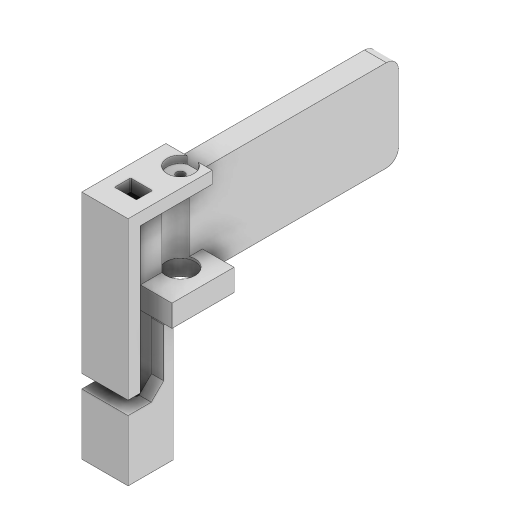
# Autodesk Inventor part: OT2-Gripper V1-1 BG Layout
Saved by Autodesk Inventor 2024.3 (Build 283343000, 343)
## iProperties
Created: 2024-09-11
Part Number: OT2-Gripper V1-1 BG Layout
Material: Generisch
Document SubType Name: Modeling
Designer: Martin
Density: 1 g/cm^3
Appearance: Vorgabe
Author: Martin
Autodesk Inventor part; units mm, degrees
ref_plane "XZ Plane" through (0, 0, 0) normal (0, 1, 0) x (-1, 0, 0)
ref_plane "XY Plane" through (0, 0, 0) normal (0, 0, 1) x (1, 0, 0)
sketch "OT2-Interface-blk" plane through (0, 0, 0) normal (0, 0, 1) x (1, 0, 0)
  circle A0 centre (25.0589, -118.2387) radius 1.5 construction
  circle A1 centre (25.0589, -91.7387) radius 1.5 construction
  circle A2 centre (-63.9411, -118.2387) radius 1.5 construction
  line L0 (32.0589, -86.2387) -> (-73.9411, -86.2387) construction
  line L1 (-73.9411, -86.2387) -> (-73.9411, -123.7387) construction
  line L2 (-73.9411, -123.7387) -> (32.0589, -123.7387) construction
  line L3 (32.0589, -123.7387) -> (32.0589, -86.2387) construction
  point P0 (-34.6142, -114.104)
  dimension "d0" = 37.5
  dimension "d1" = 26.5
  dimension "d2" = 3
  dimension "d3" = 5.5
  dimension "d4" = 7
  dimension "d5" = 89
  dimension "d6" = 106
  measures "d0" distance of L2.end L0.start
  measures "d1" distance of A0.centre A1.centre
  measures "d2" diameter of A0
  measures "d3" distance from line of L0 A1.centre
  measures "d4" distance from line of L3 A1.centre
  measures "d5" distance of A2.centre A0.centre
  measures "d6" distance of L0.start L0.end
sketch "NEMA08-04LA captive linear actor-blk" plane through (0, 0, 0) normal (0, 0, 1) x (1, 0, 0)
  line L0 (156.7218, 142.634) -> (136.7218, 142.634)
  line L1 (136.7218, 142.634) -> (136.7218, 170.634)
  line L2 (136.7218, 170.634) -> (156.7218, 170.634)
  line L3 (156.7218, 170.634) -> (156.7218, 142.634)
  line L4 (154.7218, 170.634) -> (138.7218, 170.634)
  line L5 (138.7218, 170.634) -> (138.7218, 172.134)
  line L6 (138.7218, 172.134) -> (154.7218, 172.134)
  line L7 (154.7218, 172.134) -> (154.7218, 170.634)
  line L8 (148.2218, 248.634) -> (145.2218, 248.634) construction
  line L9 (145.2218, 248.634) -> (145.2218, 252.634) construction
  line L10 (145.2218, 252.634) -> (148.2218, 252.634) construction
  line L11 (148.2218, 252.634) -> (148.2218, 248.634) construction
  line L12 (149.9718, 210.634) -> (143.4718, 210.634)
  line L13 (143.4718, 210.634) -> (143.4718, 248.634) construction
  line L14 (143.4718, 248.634) -> (149.9718, 248.634) construction
  line L15 (149.9718, 248.634) -> (149.9718, 210.634) construction
  line L16 (148.7218, 142.634) -> (144.7218, 142.634) construction
  line L17 (144.7218, 142.634) -> (144.7218, 115.634) construction
  line L18 (144.7218, 115.634) -> (148.7218, 115.634) construction
  line L19 (148.7218, 115.634) -> (148.7218, 142.634) construction
  line L20 (146.7218, 115.634) -> (146.7218, 252.634)
  line L21 (153.2218, 172.134) -> (140.2218, 172.134)
  line L22 (140.2218, 172.134) -> (140.2218, 178.134)
  line L23 (140.2218, 178.134) -> (153.2218, 178.134)
  line L24 (153.2218, 178.134) -> (153.2218, 172.134)
  line L25 (151.7218, 178.134) -> (141.7218, 178.134)
  line L26 (141.7218, 178.134) -> (141.7218, 210.634)
  line L27 (141.7218, 210.634) -> (151.7218, 210.634)
  line L28 (151.7218, 210.634) -> (151.7218, 178.134)
  line L29 (148.2218, 210.634) -> (145.2218, 210.634)
  line L30 (145.2218, 210.634) -> (145.2218, 214.634)
  line L31 (145.2218, 214.634) -> (148.2218, 214.634)
  line L32 (148.2218, 214.634) -> (148.2218, 210.634)
  line L33 (156.7218, 460.634) -> (136.7218, 460.634)
  line L34 (136.7218, 460.634) -> (136.7218, 480.634)
  line L35 (136.7218, 480.634) -> (156.7218, 480.634)
  line L36 (156.7218, 480.634) -> (156.7218, 460.634)
  circle A0 centre (154.7218, 462.634) radius 1 construction
  circle A1 centre (154.7218, 478.634) radius 1 construction
  circle A2 centre (138.7218, 478.634) radius 1 construction
  circle A3 centre (138.7218, 462.634) radius 1 construction
  circle A4 centre (146.7218, 470.634) radius 6.5
  circle A5 centre (146.7218, 470.634) radius 5
  circle A6 centre (146.7218, 470.634) radius 3.25 construction
  circle A7 centre (146.7218, 470.634) radius 1.5
  circle A8 centre (146.7218, 470.634) radius 2 construction
  circle A9 centre (146.7218, 470.634) radius 8
  line L37 (154.7218, 170.634) -> (154.7218, 167.634) construction
  line L38 (138.7218, 170.634) -> (138.7218, 167.634) construction
  point P0 (146.7218, 170.634)
  point P1 (146.7218, 210.634)
  point P2 (146.7218, 172.134)
  point P3 (146.7218, 178.134)
  point P4 (146.7218, 214.634)
  point P5 (146.7218, 480.634)
  point P6 (156.7218, 470.634)
  dimension "d9" = 4
  dimension "d10" = 16
  dimension "d11" = 1.5
  dimension "d12" = 7.5
  dimension "d14" = 3
  dimension "d15" = 6.5
  dimension "d16" = 40
  dimension "d17" = 10
  dimension "d18" = 38
  dimension "d19" = 20
  dimension "d20" = 28
  dimension "d21" = 4
  dimension "d22" = 27
  dimension "d23" = 2
  dimension "d24" = 16
  dimension "d25" = 16
  dimension "d26" = 2
  dimension "d27" = 2
  dimension "d28" = 300
  dimension "d29" = 3
  dimension "d30" = 13
  measures "d9" distance of L10.end L8.start
  measures "d10" distance of L4.start L4.end
  measures "d11" distance of L6.end L4.start
  measures "d12" distance between parallel lines of L2 L23
  measures "d14" distance of L9.end L10.end
  measures "d15" distance between parallel lines of L13 L15
  measures "d16" distance between parallel lines of L2 L27
  measures "d17" distance between parallel lines of L26 L28
  measures "d18" distance between parallel lines of L27 L14
  measures "d19" distance of L1.end L2.end
  measures "d20" distance of L2.end L0.start
  measures "d21" distance of L17.end L18.end
  measures "d22" distance of L18.end L16.start
  measures "d23" diameter of A1
  measures "d24" distance of A1.centre A0.centre
  measures "d25" distance of A1.centre A2.centre
  measures "d26" distance from line of L36 A1.centre
  measures "d27" distance from line of A1.centre L35
  measures "d28" distance from line of L2 A4.centre
  measures "d29" distance of L37.start L37.end
  measures "d30" distance between parallel lines of L22 L24
sketch "linear gudance Type10mm-blk" plane through (0, 0, 0) normal (0, 0, 1) x (1, 0, 0)
  line L0 (-133.9665, -98.7965) -> (-140.5665, -98.7965)
  line L1 (-140.5665, -98.7965) -> (-140.5665, -3.7965)
  line L2 (-140.5665, -3.7965) -> (-133.9665, -3.7965)
  line L3 (-133.9665, -3.7965) -> (-133.9665, -98.7965)
  line L4 (-135.3665, -71.2965) -> (-143.9665, -71.2965)
  line L5 (-143.9665, -71.2965) -> (-143.9665, -31.2965)
  line L6 (-143.9665, -31.2965) -> (-135.3665, -31.2965)
  line L7 (-135.3665, -31.2965) -> (-135.3665, -71.2965)
  line L8 (-135.3665, 238.7035) -> (-143.9665, 238.7035)
  line L9 (-143.9665, 238.7035) -> (-143.9665, 258.7035)
  line L10 (-143.9665, 258.7035) -> (-135.3665, 258.7035)
  line L11 (-135.3665, 258.7035) -> (-135.3665, 238.7035)
  line L12 (-133.9665, 244.2035) -> (-140.5665, 244.2035)
  line L13 (-140.5665, 244.2035) -> (-140.5665, 253.2035)
  line L14 (-140.5665, 253.2035) -> (-133.9665, 253.2035)
  line L15 (-133.9665, 253.2035) -> (-133.9665, 244.2035)
  line L16 (-423.9665, -71.2965) -> (-443.9665, -71.2965)
  line L17 (-443.9665, -71.2965) -> (-443.9665, -31.2965)
  line L18 (-443.9665, -31.2965) -> (-423.9665, -31.2965)
  line L19 (-423.9665, -31.2965) -> (-423.9665, -71.2965)
  line L20 (-429.4665, -98.7965) -> (-438.4665, -98.7965)
  line L21 (-438.4665, -98.7965) -> (-438.4665, -3.7965)
  line L22 (-438.4665, -3.7965) -> (-429.4665, -3.7965)
  line L23 (-429.4665, -3.7965) -> (-429.4665, -98.7965)
  line L24 (-433.9665, -98.7965) -> (-433.9665, -3.7965) construction
  line L25 (-135.3665, 248.7035) -> (-140.5665, 248.7035) construction
  line L26 (-133.9665, -91.2965) -> (-140.5665, -91.2965) construction
  line L27 (-136.5665, -94.2965) -> (-136.5665, -88.2965) construction
  line L28 (-136.5665, -89.4965) -> (-133.9665, -89.4965) construction
  line L29 (-133.9665, -93.0965) -> (-136.5665, -93.0965) construction
  line L30 (-136.5665, -94.2965) -> (-140.5665, -94.2965) construction
  line L31 (-136.5665, -88.2965) -> (-140.5665, -88.2965) construction
  line L32 (-136.5665, -69.4965) -> (-133.9665, -69.4965) construction
  line L33 (-133.9665, -73.0965) -> (-136.5665, -73.0965) construction
  line L34 (-136.5665, -74.2965) -> (-136.5665, -68.2965) construction
  line L35 (-133.9665, -71.2965) -> (-140.5665, -71.2965) construction
  line L36 (-136.5665, -74.2965) -> (-140.5665, -74.2965) construction
  line L37 (-136.5665, -68.2965) -> (-140.5665, -68.2965) construction
  line L38 (-136.5665, -49.4965) -> (-133.9665, -49.4965) construction
  line L39 (-133.9665, -53.0965) -> (-136.5665, -53.0965) construction
  line L40 (-136.5665, -54.2965) -> (-136.5665, -48.2965) construction
  line L41 (-133.9665, -51.2965) -> (-140.5665, -51.2965) construction
  line L42 (-136.5665, -54.2965) -> (-140.5665, -54.2965) construction
  line L43 (-136.5665, -48.2965) -> (-140.5665, -48.2965) construction
  line L44 (-136.5665, -29.4965) -> (-133.9665, -29.4965) construction
  line L45 (-133.9665, -33.0965) -> (-136.5665, -33.0965) construction
  line L46 (-136.5665, -34.2965) -> (-136.5665, -28.2965) construction
  line L47 (-133.9665, -31.2965) -> (-140.5665, -31.2965) construction
  line L48 (-136.5665, -34.2965) -> (-140.5665, -34.2965) construction
  line L49 (-136.5665, -28.2965) -> (-140.5665, -28.2965) construction
  line L50 (-136.5665, -9.4965) -> (-133.9665, -9.4965) construction
  line L51 (-133.9665, -13.0965) -> (-136.5665, -13.0965) construction
  line L52 (-136.5665, -14.2965) -> (-136.5665, -8.2965) construction
  line L53 (-133.9665, -11.2965) -> (-140.5665, -11.2965) construction
  line L54 (-136.5665, -14.2965) -> (-140.5665, -14.2965) construction
  line L55 (-136.5665, -8.2965) -> (-140.5665, -8.2965) construction
  circle A0 centre (-433.9665, -91.2965) radius 3 construction
  circle A1 centre (-433.9665, -91.2965) radius 1.8 construction
  circle A2 centre (-433.9665, -71.2965) radius 1.8 construction
  circle A3 centre (-433.9665, -71.2965) radius 3 construction
  circle A4 centre (-433.9665, -51.2965) radius 1.8 construction
  circle A5 centre (-433.9665, -51.2965) radius 3 construction
  circle A6 centre (-433.9665, -31.2965) radius 1.8 construction
  circle A7 centre (-433.9665, -31.2965) radius 3 construction
  circle A8 centre (-433.9665, -11.2965) radius 1.8 construction
  circle A9 centre (-433.9665, -11.2965) radius 3 construction
  line L56 (-140.5665, 245.7035) -> (-136.5665, 245.7035) construction
  line L57 (-136.5665, 245.7035) -> (-136.5665, 251.7035) construction
  line L58 (-136.5665, 251.7035) -> (-140.5665, 251.7035) construction
  line L59 (-136.5665, 250.5035) -> (-133.9665, 250.5035) construction
  line L60 (-133.9665, 246.9035) -> (-136.5665, 246.9035) construction
  line L61 (-143.9665, 241.2035) -> (-139.9665, 241.2035) construction
  line L62 (-143.9665, 256.2035) -> (-139.9665, 256.2035) construction
  line L63 (-143.9665, -59.2965) -> (-139.9665, -59.2965) construction
  line L64 (-143.9665, -43.2965) -> (-139.9665, -43.2965) construction
  circle A10 centre (-426.4665, -59.2965) radius 1.5 construction
  circle A11 centre (-426.4665, -43.2965) radius 1.5 construction
  circle A12 centre (-441.4665, -59.2965) radius 1.5 construction
  circle A13 centre (-441.4665, -43.2965) radius 1.5 construction
  point P0 (-136.5665, -91.2965)
  point P1 (-136.5665, -71.2965)
  point P2 (-136.5665, -51.2965)
  point P3 (-136.5665, -31.2965)
  point P4 (-136.5665, -11.2965)
  point P5 (-135.3665, -51.2965)
  point P6 (-433.9665, -31.2965)
  dimension "LgGuideHolePitch" = 20
  dimension "LgGuideLength" = 95
  dimension "LgGuideHoleDm2" = 3.6
  dimension "LgGuideHoleDm1" = 6
  dimension "LgGuideHoleDm1Depth" = 4
  dimension "LgGuideHeigth" = 6.6
  dimension "LgSystemHeigth" = 10
  dimension "LgStageHeigth" = 8.6
  dimension "LgStageLength" = 40
  dimension "LgGuideWidth" = 9
  dimension "LgStageWidth" = 20
  dimension "d48" = 300
  dimension "d49" = 300
  dimension "d52" = 20
  dimension "d57" = 3.6
  dimension "LgStageHolePitchX" = 15
  dimension "LgStageHolePitchZ" = 16
  dimension "d60" = 15
  dimension "LgStageHoleDepth" = 4
  dimension "LgStageHoleDm" = 3
  measures "LgGuideHolePitch" distance of L28.end L32.end
  measures "LgGuideLength" distance of L2.end L0.start
  measures "LgGuideHoleDm2" distance between parallel lines of L28 L29
  measures "LgGuideHoleDm1" distance of L27.start L27.end
  measures "LgGuideHoleDm1Depth" distance of L27.end L31.end
  measures "LgGuideHeigth" distance of L0.start L0.end
  measures "LgSystemHeigth" distance between parallel lines of L5 L3
  measures "LgStageHeigth" distance of L4.start L4.end
  measures "LgStageLength" distance of L4.end L5.end
  measures "LgGuideWidth" distance of L14.end L12.start
  measures "LgStageWidth" distance of L8.end L9.end
  measures "d48" distance from line of L41.start L25
  measures "d49" distance between parallel lines of L3 L24
  measures "d52" distance of A1.centre A2.centre
  measures "d57" distance between parallel lines of L59 L60
  measures "LgStageHolePitchX" distance between parallel lines of L62 L61
  measures "LgStageHolePitchZ" distance between parallel lines of L64 L63
  measures "d60" distance of point (-441.466, -43.296) point (-426.466, -43.296)
  measures "LgStageHoleDepth" distance of L63.start L63.end
  measures "LgStageHoleDm" diameter of A10
sketch "Skizze1" plane through (0, 0, 0) normal (1, 0, 0) x (0, 1, 0)
  line L0 (48, -18.75) -> (-53, -18.75)
  line L1 (-53, -18.75) -> (-53, 18.75)
  line L2 (-53, 18.75) -> (48, 18.75)
  line L3 (53, 13.75) -> (53, -13.75)
  arc A0 (53, 13.75) -> (48, 18.75) centre (48, 13.75) ccw
  arc A1 (48, -18.75) -> (53, -13.75) centre (48, -13.75) ccw
  circle A2 centre (46, 13.25) radius 2.05
  circle A3 centre (46, -13.25) radius 2.05
  circle A4 centre (-43, -13.25) radius 2.05
  line L4 (-49.5, -68.75) -> (-68, -68.75)
  line L5 (-68, -68.75) -> (-68, -43.75)
  line L6 (-68, -43.75) -> (-49.5, -43.75)
  line L7 (-49.5, -43.75) -> (-49.5, -68.75)
  line L8 (-49.5, -43.75) -> (-53.4, -43.75)
  line L9 (-53.4, -43.75) -> (-53.4, -18.75)
  line L10 (-53.4, -18.75) -> (-49.5, -18.75)
  line L11 (-49.5, -18.75) -> (-49.5, -43.75)
  line L12 (-63, -38.25) -> (-68, -38.25)
  line L13 (-68, -38.25) -> (-68, 21.25)
  line L14 (-68, 21.25) -> (-63, 21.25)
  line L15 (-63, 21.25) -> (-63, -38.25)
  line L16 (-68, 21.25) -> (-33.5, 21.25)
  line L17 (-33.5, 21.25) -> (-33.5, 26.25)
  line L18 (-33.5, 26.25) -> (-68, 26.25)
  line L19 (-68, 26.25) -> (-68, 21.25)
  line L20 (-63, 1.75) -> (-68, 1.75) construction
  line L21 (-65.5, 1.75) -> (-65.5, -38.25) construction
  line L22 (-27.5, -18.75) -> (-27.5, -9.75)
  line L23 (-27.5, -9.75) -> (-53, -9.75)
  line L24 (-38.5, -18.75) -> (-30.5, -18.75)
  line L25 (-30.5, -18.75) -> (-30.5, -9.75)
  line L26 (-30.5, -9.75) -> (-38.5, -9.75)
  line L27 (-38.5, -9.75) -> (-38.5, -18.75)
  line L28 (-65.5, -26.25) -> (-68, -26.25) construction
  line L29 (-65.5, -10.25) -> (-68, -10.25) construction
  line L30 (-53.4, -38.6642) -> (-58.4858, -43.75)
  line L31 (-63, -38.25) -> (-54.4, -38.25) construction
  line L32 (-54.4, -38.25) -> (-54.4, -27.75) construction
  circle A5 centre (-54.4, -38.25) radius 1 construction
  circle A6 centre (46, -13.25) radius 1.5 construction
  circle A7 centre (46, 13.25) radius 1.5 construction
  circle A8 centre (-43, -13.25) radius 1.5 construction
  line L33 (53, 18.75) -> (-53, 18.75) construction
  line L34 (-53, 18.75) -> (-53, -18.75) construction
  line L35 (-53, -18.75) -> (53, -18.75) construction
  line L36 (53, -18.75) -> (53, 18.75) construction
  line L37 (-28.5, -46.75) -> (-48.5, -46.75)
  line L38 (-48.5, -46.75) -> (-48.5, -18.75)
  line L39 (-48.5, -18.75) -> (-28.5, -18.75)
  line L40 (-28.5, -18.75) -> (-28.5, -46.75)
  line L41 (-30.5, -18.75) -> (-46.5, -18.75)
  line L42 (-46.5, -18.75) -> (-46.5, -17.25)
  line L43 (-46.5, -17.25) -> (-30.5, -17.25)
  line L44 (-30.5, -17.25) -> (-30.5, -18.75)
  line L45 (-37, 59.25) -> (-40, 59.25) construction
  line L46 (-40, 59.25) -> (-40, 63.25) construction
  line L47 (-40, 63.25) -> (-37, 63.25) construction
  line L48 (-37, 63.25) -> (-37, 59.25) construction
  line L49 (-35.25, 21.25) -> (-41.75, 21.25)
  line L50 (-41.75, 21.25) -> (-41.75, 59.25) construction
  line L51 (-41.75, 59.25) -> (-35.25, 59.25) construction
  line L52 (-35.25, 59.25) -> (-35.25, 21.25) construction
  line L53 (-36.5, -46.75) -> (-40.5, -46.75) construction
  line L54 (-40.5, -46.75) -> (-40.5, -73.75) construction
  line L55 (-40.5, -73.75) -> (-36.5, -73.75) construction
  line L56 (-36.5, -73.75) -> (-36.5, -46.75) construction
  line L57 (-38.5, -73.75) -> (-38.5, 63.25)
  line L58 (-32, -17.25) -> (-45, -17.25)
  line L59 (-45, -17.25) -> (-45, -11.25)
  line L60 (-45, -11.25) -> (-32, -11.25)
  line L61 (-32, -11.25) -> (-32, -17.25)
  line L62 (-33.5, -11.25) -> (-43.5, -11.25)
  line L63 (-43.5, -11.25) -> (-43.5, 21.25)
  line L64 (-43.5, 21.25) -> (-33.5, 21.25)
  line L65 (-33.5, 21.25) -> (-33.5, -11.25)
  line L66 (-37, 21.25) -> (-40, 21.25)
  line L67 (-40, 21.25) -> (-40, 25.25)
  line L68 (-40, 25.25) -> (-37, 25.25)
  line L69 (-37, 25.25) -> (-37, 21.25)
  line L70 (-28.5, 271.25) -> (-48.5, 271.25)
  line L71 (-48.5, 271.25) -> (-48.5, 291.25)
  line L72 (-48.5, 291.25) -> (-28.5, 291.25)
  line L73 (-28.5, 291.25) -> (-28.5, 271.25)
  circle A9 centre (-30.5, 273.25) radius 1 construction
  circle A10 centre (-30.5, 289.25) radius 1 construction
  circle A11 centre (-46.5, 289.25) radius 1 construction
  circle A12 centre (-46.5, 273.25) radius 1 construction
  circle A13 centre (-38.5, 281.25) radius 6.5
  circle A14 centre (-38.5, 281.25) radius 5
  circle A15 centre (-38.5, 281.25) radius 3.25 construction
  circle A16 centre (-38.5, 281.25) radius 1.5
  circle A17 centre (-38.5, 281.25) radius 2 construction
  circle A18 centre (-38.5, 281.25) radius 8
  line L74 (-30.5, -18.75) -> (-30.5, -21.75) construction
  line L75 (-46.5, -18.75) -> (-46.5, -21.75) construction
  line L76 (-53, -55.25) -> (-59.6, -55.25)
  line L77 (-59.6, -55.25) -> (-59.6, 39.75)
  line L78 (-59.6, 39.75) -> (-53, 39.75)
  line L79 (-53, 39.75) -> (-53, -55.25)
  line L80 (-54.4, -27.75) -> (-63, -27.75)
  line L81 (-63, -27.75) -> (-63, 12.25)
  line L82 (-63, 12.25) -> (-54.4, 12.25)
  line L83 (-54.4, 12.25) -> (-54.4, -27.75)
  line L84 (-54.4, 282.25) -> (-63, 282.25)
  line L85 (-63, 282.25) -> (-63, 302.25)
  line L86 (-63, 302.25) -> (-54.4, 302.25)
  line L87 (-54.4, 302.25) -> (-54.4, 282.25)
  line L88 (-53, 287.75) -> (-59.6, 287.75)
  line L89 (-59.6, 287.75) -> (-59.6, 296.75)
  line L90 (-59.6, 296.75) -> (-53, 296.75)
  line L91 (-53, 296.75) -> (-53, 287.75)
  line L92 (-343, -27.75) -> (-363, -27.75)
  line L93 (-363, -27.75) -> (-363, 12.25)
  line L94 (-363, 12.25) -> (-343, 12.25)
  line L95 (-343, 12.25) -> (-343, -27.75)
  line L96 (-348.5, -55.25) -> (-357.5, -55.25)
  line L97 (-357.5, -55.25) -> (-357.5, 39.75)
  line L98 (-357.5, 39.75) -> (-348.5, 39.75)
  line L99 (-348.5, 39.75) -> (-348.5, -55.25)
  line L100 (-353, -55.25) -> (-353, 39.75) construction
  line L101 (-54.4, 292.25) -> (-59.6, 292.25) construction
  line L102 (-53, -47.75) -> (-59.6, -47.75) construction
  line L103 (-55.6, -50.75) -> (-55.6, -44.75) construction
  line L104 (-55.6, -45.95) -> (-53, -45.95) construction
  line L105 (-53, -49.55) -> (-55.6, -49.55) construction
  line L106 (-55.6, -50.75) -> (-59.6, -50.75) construction
  line L107 (-55.6, -44.75) -> (-59.6, -44.75) construction
  line L108 (-55.6, -25.95) -> (-53, -25.95) construction
  line L109 (-53, -29.55) -> (-55.6, -29.55) construction
  line L110 (-55.6, -30.75) -> (-55.6, -24.75) construction
  line L111 (-53, -27.75) -> (-59.6, -27.75) construction
  line L112 (-55.6, -30.75) -> (-59.6, -30.75) construction
  line L113 (-55.6, -24.75) -> (-59.6, -24.75) construction
  line L114 (-55.6, -5.95) -> (-53, -5.95) construction
  line L115 (-53, -9.55) -> (-55.6, -9.55) construction
  line L116 (-55.6, -10.75) -> (-55.6, -4.75) construction
  line L117 (-53, -7.75) -> (-59.6, -7.75) construction
  line L118 (-55.6, -10.75) -> (-59.6, -10.75) construction
  line L119 (-55.6, -4.75) -> (-59.6, -4.75) construction
  line L120 (-55.6, 14.05) -> (-53, 14.05) construction
  line L121 (-53, 10.45) -> (-55.6, 10.45) construction
  line L122 (-55.6, 9.25) -> (-55.6, 15.25) construction
  line L123 (-53, 12.25) -> (-59.6, 12.25) construction
  line L124 (-55.6, 9.25) -> (-59.6, 9.25) construction
  line L125 (-55.6, 15.25) -> (-59.6, 15.25) construction
  line L126 (-55.6, 34.05) -> (-53, 34.05) construction
  line L127 (-53, 30.45) -> (-55.6, 30.45) construction
  line L128 (-55.6, 29.25) -> (-55.6, 35.25) construction
  line L129 (-53, 32.25) -> (-59.6, 32.25) construction
  line L130 (-55.6, 29.25) -> (-59.6, 29.25) construction
  line L131 (-55.6, 35.25) -> (-59.6, 35.25) construction
  circle A19 centre (-353, -47.75) radius 3 construction
  circle A20 centre (-353, -47.75) radius 1.8 construction
  circle A21 centre (-353, -27.75) radius 1.8 construction
  circle A22 centre (-353, -27.75) radius 3 construction
  circle A23 centre (-353, -7.75) radius 1.8 construction
  circle A24 centre (-353, -7.75) radius 3 construction
  circle A25 centre (-353, 12.25) radius 1.8 construction
  circle A26 centre (-353, 12.25) radius 3 construction
  circle A27 centre (-353, 32.25) radius 1.8 construction
  circle A28 centre (-353, 32.25) radius 3 construction
  line L132 (-59.6, 289.25) -> (-55.6, 289.25) construction
  line L133 (-55.6, 289.25) -> (-55.6, 295.25) construction
  line L134 (-55.6, 295.25) -> (-59.6, 295.25) construction
  line L135 (-55.6, 294.05) -> (-53, 294.05) construction
  line L136 (-53, 290.45) -> (-55.6, 290.45) construction
  line L137 (-63, 284.75) -> (-59, 284.75) construction
  line L138 (-63, 299.75) -> (-59, 299.75) construction
  line L139 (-63, -15.75) -> (-59, -15.75) construction
  line L140 (-63, 0.25) -> (-59, 0.25) construction
  circle A29 centre (-345.5, -15.75) radius 1.5 construction
  circle A30 centre (-345.5, 0.25) radius 1.5 construction
  circle A31 centre (-360.5, -15.75) radius 1.5 construction
  circle A32 centre (-360.5, 0.25) radius 1.5 construction
  point P0 (0, 0)
  point P1 (53, 0)
  point P2 (0, -18.75)
  dimension "d89" = 27.5
  dimension "d90" = 38
  dimension "d7" = 5
  dimension "d8" = 4.1
  dimension "d76" = 25
  dimension "d78" = 3.5
  dimension "d79" = 25
  dimension "d80" = 18.5
  dimension "d81" = 8
  dimension "d82" = 1
  dimension "d83" = 8.4
  dimension "d84" = 5
  dimension "d85" = 10
  dimension "d86" = 1
  dimension "d87" = 5
  dimension "d88" = 5.5
  dimension "d91" = 10.5
  dimension "d92" = 9
  dimension "d93" = 12
  dimension "d94" = 9
  dimension "d95" = 6
  dimension "d96" = 10.5
  dimension "d97" = 10.5
  dimension "d98" = 45
  dimension "d105" = 22
  constraints: 66 end point, 12 horizontal, 12 parallel, 10 perpendicular, 8 point on line, 6 centre point, 6 tangent, 6 vertical, 4 point on circle, 3 equal radius, 2 collinear, 2 midpoint, 1 coincident, 1 horizontal alignment, 1 vertical alignment, 9 other
  measures "d7" radius of A0
  measures "d8" diameter of A2
  measures "d79" distance of L6.end L4.start
  measures "d80" distance of L4.start L4.end
  measures "d84" distance of L16.end L17.end
  measures "d87" distance between parallel lines of L13 L15
  measures "d88" distance between parallel lines of L6 L12
  measures "d94" distance of L22.start L22.end
  measures "d98" angle of L9 L30
extrude "Extrusion1" add sketch "Skizze1" along normal mid plane 19 contours L16 L69 L68 L57 L18 L17 | L57 L68 L69 L16 | L16 L67 L68 L57 | L16 L79 L18 L57 L68 L67 | L16 L77 L18 L79 | L16 L14 L19 L18 L77 | L15 L12 L13 L14
extrude "Extrusion2" add sketch "Skizze1" along normal mid plane 19 separate body contours L11 L6 L79 L0 | L79 L6 L9 L10 | L7 L4 L5 L6 L77 L76 L79 | L79 L76 L77 L6 | L9 L6 L30
extrude "Extrusion3" add sketch "Skizze1" along normal blind 9 from surface at -9.5 separate body contours L0 L22 L23 L65 L2 A0 L3 A1 | L0 L25 L23 L22 | L0 L27 L43 L25 | L25 L43 L61 L60 L65 L23 | L0 L42 L43 L27 | L65 L60 L27 L23 | L23 L57 L2 L65 | L0 L1 L23 L63 L60 L59 A4 L43 L42 | L43 L59 A4 L60 L27 | L27 L60 L61 L43 | L27 L60 A4 L63 L23 | L23 L63 L2 L57 | L23 L1 L2 L63 | L60 A4 | A4 L59 L60 | A4 L59 | L60 A4 L59 | A2 | A3
sketch "Skizze2" plane through (-0.5, -53, -18.75) normal (0, 0, -1) x (-1, 0, 0)
  line L0 (9, 101) -> (9, 0) construction
  line L1 (-13, 25.5) -> (9, 25.5)
  line L2 (9, 25.5) -> (9, 0)
  line L3 (9, 0) -> (-13, 0)
  line L4 (-13, 0) -> (-13, 25.5)
  circle A0 centre (-10, 22.5) radius 3 construction
  line L5 (-0.5, -6.6) -> (-0.5, 0) construction
  line L6 (-4.7, 0) -> (3.7, 0)
  line L7 (4, -0.3) -> (4, -6.3)
  line L8 (3.7, -6.6) -> (-4.7, -6.6)
  line L9 (-5, -6.3) -> (-5, -0.3)
  arc A1 (-5, -6.3) -> (-4.7, -6.6) centre (-4.7, -6.3) ccw
  arc A2 (3.7, -6.6) -> (4, -6.3) centre (3.7, -6.3) ccw
  arc A3 (4, -0.3) -> (3.7, 0) centre (3.7, -0.3) ccw
  arc A4 (-4.7, 0) -> (-5, -0.3) centre (-4.7, -0.3) ccw
  line L10 (8, -313.5) -> (-12, -313.5)
  line L11 (-12, -313.5) -> (-12, -285.5)
  line L12 (-12, -285.5) -> (8, -285.5)
  line L13 (8, -285.5) -> (8, -313.5)
  line L14 (6, -285.5) -> (-10, -285.5)
  line L15 (-10, -285.5) -> (-10, -284)
  line L16 (-10, -284) -> (6, -284)
  line L17 (6, -284) -> (6, -285.5)
  line L18 (-0.5, -207.5) -> (-3.5, -207.5) construction
  line L19 (-3.5, -207.5) -> (-3.5, -203.5) construction
  line L20 (-3.5, -203.5) -> (-0.5, -203.5) construction
  line L21 (-0.5, -203.5) -> (-0.5, -207.5) construction
  line L22 (1.25, -245.5) -> (-5.25, -245.5)
  line L23 (-5.25, -245.5) -> (-5.25, -207.5) construction
  line L24 (-5.25, -207.5) -> (1.25, -207.5) construction
  line L25 (1.25, -207.5) -> (1.25, -245.5) construction
  line L26 (0, -313.5) -> (-4, -313.5) construction
  line L27 (-4, -313.5) -> (-4, -340.5) construction
  line L28 (-4, -340.5) -> (0, -340.5) construction
  line L29 (0, -340.5) -> (0, -313.5) construction
  line L30 (-2, -340.5) -> (-2, -203.5)
  line L31 (4.5, -284) -> (-8.5, -284)
  line L32 (-8.5, -284) -> (-8.5, -278)
  line L33 (-8.5, -278) -> (4.5, -278)
  line L34 (4.5, -278) -> (4.5, -284)
  line L35 (3, -278) -> (-7, -278)
  line L36 (-7, -278) -> (-7, -245.5)
  line L37 (-7, -245.5) -> (3, -245.5)
  line L38 (3, -245.5) -> (3, -278)
  line L39 (-0.5, -245.5) -> (-3.5, -245.5)
  line L40 (-3.5, -245.5) -> (-3.5, -241.5)
  line L41 (-3.5, -241.5) -> (-0.5, -241.5)
  line L42 (-0.5, -241.5) -> (-0.5, -245.5)
  line L43 (8, 4.5) -> (-12, 4.5)
  line L44 (-12, 4.5) -> (-12, 24.5)
  line L45 (-12, 24.5) -> (8, 24.5)
  line L46 (8, 24.5) -> (8, 4.5)
  circle A5 centre (6, 6.5) radius 1 construction
  circle A6 centre (6, 22.5) radius 1 construction
  circle A7 centre (-10, 22.5) radius 1 construction
  circle A8 centre (-10, 6.5) radius 1 construction
  circle A9 centre (-2, 14.5) radius 6.5
  circle A10 centre (-2, 14.5) radius 5
  circle A11 centre (-2, 14.5) radius 3.25 construction
  circle A12 centre (-2, 14.5) radius 1.5
  circle A13 centre (-2, 14.5) radius 2 construction
  circle A14 centre (-2, 14.5) radius 8
  line L47 (6, -285.5) -> (6, -288.5) construction
  line L48 (-10, -285.5) -> (-10, -288.5) construction
  point P0 (-0.5, 53)
  point P1 (-0.5, 0)
  point P2 (-0.5, 0)
  point P3 (-0.5, 0)
  point P4 (-0.5, 14.5)
  point P5 (-0.5, 25.5)
  point P6 (4, -6.6)
  point P7 (-5, -6.6)
  point P8 (3.7, 0)
  point P9 (-4.7, 0)
  dimension "d106" = 1
  dimension "d120" = 9
  dimension "d121" = 0.3
  constraints: 16 end point, 10 tangent, 8 point on circle, 5 centre point, 5 point on line, 3 equal radius, 3 parallel, 2 horizontal, 2 midpoint, 2 perpendicular, 2 other
  measures "d120" distance of point (4, -6.6) point (-5, -6.6)
  measures "d121" radius of A1
extrude "Extrusion4" add sketch "Skizze2" against normal up to surface (9 mm away) contours L1 L2 L3 L4 | L43 L44 L45 L46 | A9 | A10 | A12 | A14 bodies 3
ref_plane "LinearActorReferencePlane" through (1.5, -38.5, -18.75) normal (1, 0, 0) x (0, 0, -1)
sketch "Skizze3" plane through (1.5, -38.5, -18.75) normal (1, 0, 0) x (0, 0, -1)
  line L0 (-383, 0) -> (128, 0) construction
  line L1 (0, -10) -> (0, 10) construction
  line L2 (0, 8) -> (-8, 8)
  line L3 (-8, 8) -> (-8, 0)
  line L4 (-8, 0) -> (0, 0)
  line L5 (0, 0) -> (0, 8)
  line L6 (-8, 0) -> (-40, 0)
  line L7 (-40, 0) -> (-40, 6)
  line L8 (-40, 6) -> (-8, 6)
  line L9 (-8, 6) -> (-8, 0)
  line L10 (28, 10) -> (28, -10)
  line L11 (28, -10) -> (0, -10)
  line L12 (0, -10) -> (0, 10)
  line L13 (0, 10) -> (28, 10)
  line L14 (0, 8) -> (0, -8)
  line L15 (0, -8) -> (-1.5, -8)
  line L16 (-1.5, -8) -> (-1.5, 8)
  line L17 (-1.5, 8) -> (0, 8)
  line L18 (-78, 1.5) -> (-78, -1.5) construction
  line L19 (-78, -1.5) -> (-82, -1.5) construction
  line L20 (-82, -1.5) -> (-82, 1.5) construction
  line L21 (-82, 1.5) -> (-78, 1.5) construction
  line L22 (-40, 3.25) -> (-40, -3.25)
  line L23 (-40, -3.25) -> (-78, -3.25) construction
  line L24 (-78, -3.25) -> (-78, 3.25) construction
  line L25 (-78, 3.25) -> (-40, 3.25) construction
  line L26 (28, 2) -> (28, -2) construction
  line L27 (28, -2) -> (55, -2) construction
  line L28 (55, -2) -> (55, 2) construction
  line L29 (55, 2) -> (28, 2) construction
  line L30 (55, 0) -> (-82, 0)
  line L31 (-1.5, 6.5) -> (-1.5, -6.5)
  line L32 (-1.5, -6.5) -> (-7.5, -6.5)
  line L33 (-7.5, -6.5) -> (-7.5, 6.5)
  line L34 (-7.5, 6.5) -> (-1.5, 6.5)
  line L35 (-7.5, 5) -> (-7.5, -5)
  line L36 (-7.5, -5) -> (-40, -5)
  line L37 (-40, -5) -> (-40, 5)
  line L38 (-40, 5) -> (-7.5, 5)
  line L39 (-40, 1.5) -> (-40, -1.5)
  line L40 (-40, -1.5) -> (-44, -1.5)
  line L41 (-44, -1.5) -> (-44, 1.5)
  line L42 (-44, 1.5) -> (-40, 1.5)
  line L43 (-290, 10) -> (-290, -10)
  line L44 (-290, -10) -> (-310, -10)
  line L45 (-310, -10) -> (-310, 10)
  line L46 (-310, 10) -> (-290, 10)
  circle A0 centre (-292, 8) radius 1 construction
  circle A1 centre (-308, 8) radius 1 construction
  circle A2 centre (-308, -8) radius 1 construction
  circle A3 centre (-292, -8) radius 1 construction
  circle A4 centre (-300, 0) radius 6.5
  circle A5 centre (-300, 0) radius 5
  circle A6 centre (-300, 0) radius 3.25 construction
  circle A7 centre (-300, 0) radius 1.5
  circle A8 centre (-300, 0) radius 2 construction
  circle A9 centre (-300, 0) radius 8
  line L47 (0, 8) -> (3, 8) construction
  line L48 (0, -8) -> (3, -8) construction
  point P0 (-18.75, 38.5)
  point P1 (-8, 6)
  dimension "d111" = 1
  dimension "d112" = 0.5
  constraints: 16 end point, 5 horizontal, 4 parallel, 3 vertical, 2 perpendicular
revolve "Umdrehung1" cut sketch "Skizze3" angle 360 about axis through (1.5, -38.5, -10.75) along (0, 0, -1) bodies 3 contours L5 L4 L16 L2 | L16 L34 L33 L38 L3 L2 | L16 L4 L33 L34 | L3 L38 L7 L8 | L4 L3 L38 L33 | L3 L6 L7 L38
sketch "Skizze4" plane through (-9.5, -68, 26.25) normal (0, 0, 1) x (1, 0, 0)
  arc A0 (9, 35.1569) -> (9, 23.8431) centre (11, 29.5) ccw projected
  point P0 (9.5, 68)
  constraints: 1 coincident
hole "Bohrung1" at (1.5, -38.5, 26.25) direction (0, 0, -1) diameter 3.4 end through all counterbore diameter 11 counterbore depth 3 bodies 1 clearance for "Sechskantkopfschraube ISO 24017" size "M3" standard "ISO"
extrude "Extrusion5" cut sketch "Skizze2" along normal through all both and the other way through all contours L3 A3 L7 A2 L8 A1 L9 A4 bodies 2 1
sketch "Skizze5" plane through (-9.5, -53, -18.75) normal (-1, 0, 0) x (0, 0, 1)
  point P0 (18.75, 53)
  point P1 (32, 99)
  point P2 (5.5, 99)
  point P3 (5.5, 10)
hole "Bohrung2" at (-9.5, 46, -13.25) at (-9.5, 46, 13.25) at (-9.5, -43, -13.25) direction (1, 0, 0) diameter 4.1 depth 8 counterbore diameter 5 counterbore depth 1 bodies 3
equation "\"d3\" = -0.5 * d1 + 0.5 * d0"
equation "\"d26\" = -0.5 * d25 + 0.5 * d19"
equation "\"d27\" = d26"
equation "\"d49\" = d48"
equation "\"d57\" = LgGuideHoleDm2"
equation "\"d60\" = LgStageHolePitchX"
